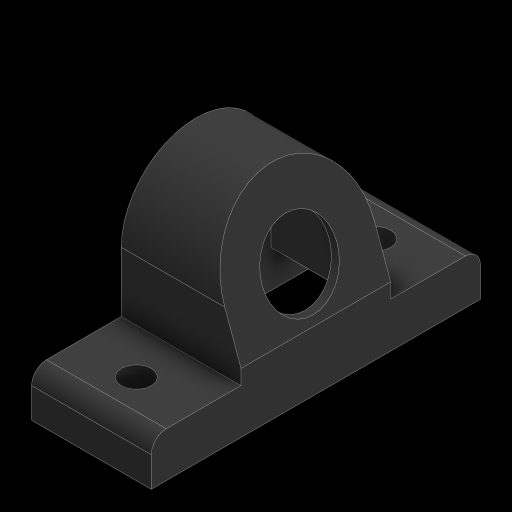
# Autodesk Inventor part: ANS12-1-BK
Saved by Autodesk Inventor 2024 (Build 280153000, 153)
## iProperties
Created: 2023-12-13
Part Number: ANS12-1-BK
Material: Rubber
Document SubType Name: Modeling
Designer: bennk
Density: 0.93 g/cm^3
Appearance: Rubber - Black
Mass: 525.317 g
Surface Area: 1850.32 cm^2
Volume: 564.857 cm^3
Author: bennk
Autodesk Inventor part; units mm, degrees
ref_plane "YZ Plane" through (0, 0, 0) normal (1, 0, 0) x (0, 1, 0)
ref_plane "XZ Plane" through (0, 0, 0) normal (0, 1, 0) x (-1, 0, 0)
ref_plane "XY Plane" through (0, 0, 0) normal (0, 0, 1) x (1, 0, 0)
sketch "Sketch1" plane through (0, 0, 0) normal (0, 1, 0) x (-1, 0, 0)
  line L0 (50.8, 139.7) -> (-50.8, 139.7)
  line L1 (-50.8, 139.7) -> (-50.8, -139.7)
  line L2 (-50.8, -139.7) -> (50.8, -139.7)
  line L3 (50.8, -139.7) -> (50.8, 139.7)
  line L4 (50.8, 139.7) -> (-50.8, -139.7) construction
  line L5 (-50.8, 139.7) -> (50.8, -139.7) construction
  point P0 (0, 0)
  dimension "d0" = 279.4
  dimension "d1" = 101.6
  constraints: 12 end point, 2 midpoint, 2 parallel, 1 horizontal, 1 perpendicular
  measures "d0" distance of L2.end L0.start
  measures "d1" distance of L1.end L2.end
extrude "BASE" add sketch "Sketch1" along normal blind 38.1
sketch "Sketch2" plane through (50.8, 0, 139.7) normal (1, 0, 0) x (0, 0, -1)
  circle A0 centre (139.7, 88.9) radius 63.5
  line L0 (76.2, 88.9) -> (203.2, 88.9)
  line L1 (203.2, 88.9) -> (203.2, 38.1)
  line L2 (203.2, 38.1) -> (76.2, 38.1)
  line L3 (76.2, 38.1) -> (76.2, 88.9)
  line L4 (0, 0) -> (279.4, 0) projected
  line L5 (0, 38.1) -> (279.4, 38.1) projected
  point P0 (139.7, 0)
  point P1 (139.7, 0)
  point P2 (139.7, 0)
  dimension "d4" = 127
  dimension "d5" = 88.9
  dimension "d7" = 0
  constraints: 8 end point, 4 midpoint, 2 parallel, 2 point on circle, 1 centre point, 1 collinear, 1 horizontal, 1 perpendicular
  measures "d4" diameter of A0
  measures "d5" distance between parallel lines of L0 L4
  measures "d7" horizontal distance of point (139.7, 0) point (139.7, 88.9)
extrude "ARCH" add sketch "Sketch2" against normal blind 101.6 contours L0 A0 | L1 L2 A0 | A0 L2 L0 | A0 L2 L3
sketch "Sketch3" plane through (-50.8, 0, 139.7) normal (0, 0, 1) x (1, 0, 0)
  line L0 (101.6, 0) -> (101.6, 38.1) projected
  line L1 (64.6206, 152.4) -> (101.6, 152.4)
  line L2 (101.6, 152.4) -> (101.6, 50.8)
  line L3 (101.6, 38.1) -> (101.6, 88.9) projected
  line L4 (101.6, 50.8) -> (64.6206, 152.4)
  line L5 (101.6, 50.8) -> (101.6, 50.8)
  line L6 (0, 0) -> (101.6, 0) projected
  line L7 (101.6, 88.9) -> (101.6, 152.4) projected
  point P0 (50.8, 0)
  point P1 (101.6, 50.8)
  dimension "d11" = 50.8
  dimension "d12" = 20
  constraints: 8 end point, 2 perpendicular, 2 point on line, 1 collinear
  measures "d11" distance between parallel lines of L6 L5
  measures "d12" angle of L7 L4
extrude "ANGLED CUT" cut sketch "Sketch3" against normal through all
sketch "Sketch4" plane through (0, 38.1, 0) normal (0, 1, 0) x (1, 0, 0)
  line L0 (-50.8, 139.7) -> (-50.8, 63.5) projected
  point P0 (0, 0)
  point P1 (0, 101.6)
  dimension "d22" = 101.6
  dimension "d23" = 50.8
  measures "d22" distance of point (0, 0) point (0, 101.6)
  measures "d23" distance from line of L0 point (0, 101.6)
hole "Hole1" at (0, 38.1, -101.6) direction (0, -1, 0) diameter 25.4 end through all
mirror "Mirror1" about plane through (0, 0, 0) normal (0, 0, 1) of "ANGLED CUT", "Hole1"
fillet "Fillet1" radius 12.7 2 edges at (0, 38.1, 139.7) (0, 38.1, -139.7)
shell "Shell1" thickness 6.35 removed faces 1 at (37.3506, 0, -31.4619)
sketch "Sketch5" plane through (50.8, 0, 139.7) normal (1, 0, 0) x (0, 0, -1)
  circle A0 centre (139.7, 88.9) radius 31.75
  line L0 (0, 0) -> (279.4, 0) projected
  point P0 (139.7, 0)
  point P1 (139.7, 0)
  dimension "d26" = 63.5
  dimension "d27" = 88.9
  dimension "d28" = 0
  constraints: 1 centre point, 1 midpoint
  measures "d26" diameter of A0
  measures "d27" distance from line of L0 A0.centre
  measures "d28" horizontal distance of point (139.7, 0) A0.centre
extrude "Extrusion4" cut sketch "Sketch5" along normal up to surface surface through (44.833, 48.6282, 139.7) normal (-0.9396926, -0.3420201, 0)
body "Solid1"
